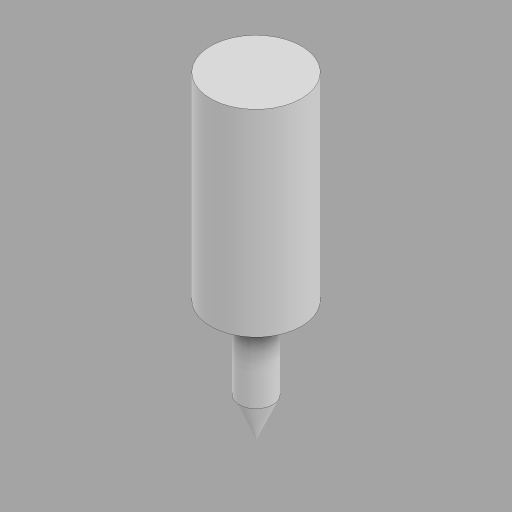
# Autodesk Inventor part: pen
Saved by Autodesk Inventor 2023.1 (Build 271208000, 208)
## iProperties
Created: 2022-10-29
Part Number: pen
Material: 일반
Document SubType Name: Modeling
Designer: 박동준
Density: 1 g/cm^3
Appearance: 기본값
Author: 박동준
Autodesk Inventor part; units mm, degrees
ref_plane "YZ Plane" through (0, 0, 0) normal (1, 0, 0) x (0, 1, 0)
ref_plane "XZ Plane" through (0, 0, 0) normal (0, 1, 0) x (-1, 0, 0)
ref_plane "XY Plane" through (0, 0, 0) normal (0, 0, 1) x (1, 0, 0)
sketch "스케치1" plane through (0, 0, 0) normal (0, 0, 1) x (1, 0, 0)
  line L0 (0, 14.9) -> (0, -14.9)
  line L1 (3, -4.2604) -> (1.5, -4.2604)
  line L2 (1.5, -4.2604) -> (1.5, -11.4821)
  line L3 (1.5, -11.4821) -> (0, -14.9)
  line L4 (3, -4.2604) -> (4, -4.2604)
  line L5 (0, 13.1) -> (4, 13.1)
  line L6 (4, 13.1) -> (4, -4.2604)
  point P0 (0, 0)
  point P1 (0, 0)
  point P2 (4, 0)
  point P3 (4, 4.4198)
  dimension "d3" = 1.5
  dimension "d5" = 1.5
  dimension "d8" = 14.9
  dimension "d10" = 3.7326
  dimension "d12" = 28
  dimension "d13" = 4
  dimension "d14" = 8.6802
  constraints: 14 end point, 3 horizontal, 2 coincident, 2 midpoint, 2 perpendicular, 1 horizontal alignment, 1 point on line, 1 vertical
  measures "d3" horizontal distance of L0.end L2.end
  measures "d5" distance of L1.start L1.end
  measures "d8" vertical distance of point (4, 0) L0.end
  measures "d10" distance of L2.end L0.end
  measures "d12" distance from line of L5 L0.end
  measures "d13" distance of L5.start L5.end
  measures "d14" distance from line of point (4, 4.42) L1
revolve "회전1" add sketch "스케치1" angle 360 about axis through (0, 14.9, 0) along (0, -1, 0)
